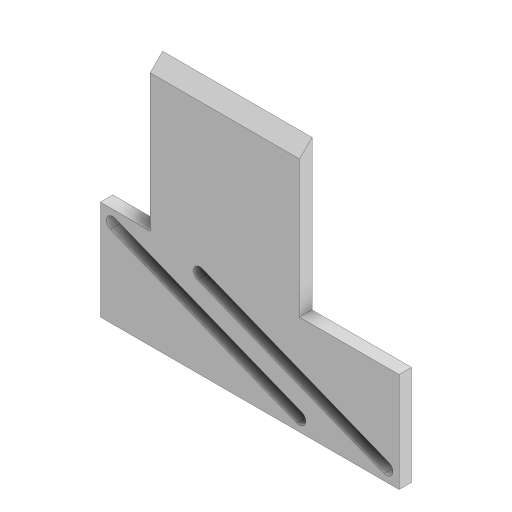
# Autodesk Inventor part: Tall Wall Lift
Saved by Autodesk Inventor 2024.2 (Build 282272000, 272)
## iProperties
Created: 2024-12-02
Part Number: Tall Wall Lift
Material: Generic
Document SubType Name: Modeling
Designer: rhond
Density: 1 g/cm^3
Appearance: Default
Author: rhond
Autodesk Inventor part; units mm, degrees
ref_plane "YZ Plane" through (0, 0, 0) normal (1, 0, 0) x (0, 1, 0)
ref_plane "XZ Plane" through (0, 0, 0) normal (0, 1, 0) x (-1, 0, 0)
ref_plane "XY Plane" through (0, 0, 0) normal (0, 0, 1) x (1, 0, 0)
sketch "Sketch1" plane through (0, 0, 0) normal (0, 0, 1) x (1, 0, 0)
  line L0 (-29.0928, 7.1512) -> (47.1072, 7.1512)
  line L1 (47.1072, 7.1512) -> (47.1072, 83.3512)
  line L2 (47.1072, 83.3512) -> (-29.0928, 83.3512)
  line L3 (-29.0928, 83.3512) -> (-29.0928, 7.1512)
  line L4 (-54.4928, 7.1512) -> (97.9072, 7.1512)
  line L5 (97.9072, 7.1512) -> (97.9072, -43.6488)
  line L6 (97.9072, -43.6488) -> (-54.4928, -43.6488)
  line L7 (-54.4928, -43.6488) -> (-54.4928, 7.1512)
  circle A0 centre (-48.1428, 0.8012) radius 3.175
  circle A1 centre (47.1072, -37.2988) radius 3.175
  line L8 (-46.9636, 3.7491) -> (48.2864, -34.3509)
  line L9 (-49.322, -2.1467) -> (45.928, -40.2467)
  circle A2 centre (-3.6928, 0.8012) radius 3.175
  line L10 (-4.872, -2.1467) -> (90.378, -40.2467)
  line L11 (-2.5136, 3.7491) -> (92.7364, -34.3509)
  circle A3 centre (91.5572, -37.2988) radius 3.175
  point P0 (0, 0)
  point P1 (-29.0928, 7.1512)
  dimension "d0" = 76.2
  dimension "d1" = 76.2
  dimension "d2" = 152.4
  dimension "d3" = 50.8
  dimension "d4" = 25.4
  dimension "d5" = 6.35
  dimension "d6" = 6.35
  dimension "d7" = 6.35
  dimension "d8" = 6.35
  dimension "d9" = 6.35
  dimension "d10" = 6.35
  dimension "d11" = 6.35
  dimension "d12" = 6.35
  constraints: 24 end point, 8 point on circle, 6 tangent, 4 centre point, 4 parallel, 3 horizontal, 2 perpendicular, 1 point on line
  measures "d0" distance of L3.start L1.end
  measures "d1" distance of L1.end L1.start
  measures "d2" distance of L5.end L6.end
  measures "d3" distance of L6.end L4.start
  measures "d4" distance between parallel lines of L7 L3
  measures "d5" diameter of A0
  measures "d6" distance from line of L4 A0.centre
  measures "d7" distance from line of L7 A0.centre
  measures "d8" diameter of A1
  measures "d9" distance from line of L6 A1.centre
  measures "d10" diameter of A2
  measures "d11" diameter of A3
  measures "d12" distance from line of L5 A3.centre
extrude "Extrusion1" add sketch "Sketch1" along normal blind 6.35
chamfer "Chamfer1" distance 6.35 angle 45 1 edges at (9.0072, 83.3512, 6.35)
body "Solid1"
